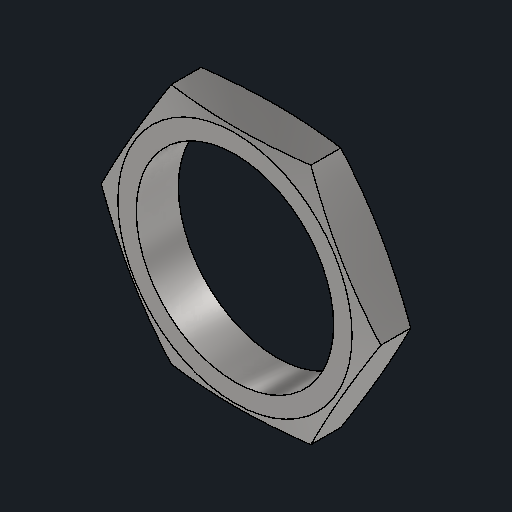
# Autodesk Inventor part: Nut
Saved by Autodesk Inventor 2026.2 (Build 302298000, 298)
## iProperties
Created: 2015-04-29
Part Number: Nut
Material: Stainless Steel
Document SubType Name: Modeling
Designer: Philip
Density: 8 g/cm^3
Appearance: Semi-Polished
Author: Philip
Autodesk Inventor part; units mm, degrees
ref_plane "YZ Plane" through (0, 0, 0) normal (1, 0, 0) x (0, 1, 0)
ref_plane "XZ Plane" through (0, 0, 0) normal (0, 1, 0) x (-1, 0, 0)
ref_plane "XY Plane" through (0, 0, 0) normal (0, 0, 1) x (1, 0, 0)
sketch "Sketch1" plane through (0, 0, 0) normal (0, 0, 1) x (1, 0, 0)
  line L0 (-3.3729, 5.842) -> (3.3729, 5.842)
  line L1 (3.3729, 5.842) -> (6.7458, 0)
  line L2 (6.7458, 0) -> (3.3729, -5.842)
  line L3 (3.3729, -5.842) -> (-3.3729, -5.842)
  line L4 (-3.3729, -5.842) -> (-6.7458, 0)
  line L5 (-6.7458, 0) -> (-3.3729, 5.842)
  point P0 (0, 0)
  point P1 (0, 0)
  dimension "d0" = 11.684
  constraints: 12 end point, 1 coincident, 1 horizontal, 13 other
  measures "d0" distance between parallel lines of L0 L3
extrude "Extrusion1" add sketch "Sketch1" along normal mid plane 2.032
sketch "Sketch2" plane through (0, 0, 0) normal (1, 0, 0) x (0, 1, 0)
  line L0 (5.6521, 1.016) -> (7.9534, 1.016)
  line L1 (7.9534, 1.016) -> (7.9534, 0.3994)
  line L2 (7.9534, 0.3994) -> (5.6521, 1.016)
  line L3 (0, 1.016) -> (5.842, 1.016) projected
  line L4 (0, -0.4064) -> (0, 2.4384) projected
  point P0 (0, 0)
  dimension "d3" = 15
  constraints: 6 end point, 1 collinear, 1 horizontal, 1 perpendicular
  measures "d3" angle of L2 L0
revolve "Revolution1" cut sketch "Sketch2" angle 360 about axis through (0, 0, -10) along (0, 0, 1)
mirror "Mirror1" about plane through (0, 0, 0) normal (0, 0, 1) of "Revolution1"
hole "Hole1" at (0, 0, 1.016) direction (0, 0, -1) diameter 9.525 end through all
body "Solid1"
